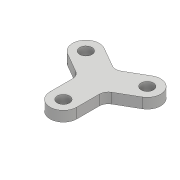
# Autodesk Inventor part: carrier2
Saved by Autodesk Inventor 2018 (Build 220112000, 112)
## iProperties
Created: 2019-12-31
Part Number: carrier2
Material: 一般
Document SubType Name: Modeling
Designer: louis
Density: 1 g/cm^3
Appearance: 預設
Author: louis
Autodesk Inventor part; units mm, degrees
ref_plane "YZ Plane" through (0, 0, 0) normal (1, 0, 0) x (0, 1, 0)
ref_plane "XZ Plane" through (0, 0, 0) normal (0, 1, 0) x (-1, 0, 0)
ref_plane "XY Plane" through (0, 0, 0) normal (0, 0, 1) x (1, 0, 0)
sketch "草圖1" plane through (0, 0, 0) normal (0, 0, 1) x (1, 0, 0)
  line L0 (0, 0) -> (-29.8779, 17.25) construction
  line L1 (0, 0) -> (0, -34.5) construction
  circle A0 centre (29.8779, 17.25) radius 6
  circle A1 centre (0, -34.5) radius 6
  circle A2 centre (-29.8779, 17.25) radius 6
  line L2 (-23.3779, 28.5083) -> (-4.3253, 17.5083)
  arc A3 (-4.3253, 17.5083) -> (4.3253, 17.5083) centre (0, 25) ccw
  line L3 (4.3253, 17.5083) -> (23.3779, 28.5083)
  line L4 (23.3779, 28.5083) -> (23.3779, 28.5083)
  arc A4 (36.3779, 5.9917) -> (23.3779, 28.5083) centre (29.8779, 17.25) ccw
  line L5 (36.3779, 5.9917) -> (17.3253, -5.0083)
  arc A5 (17.3253, -5.0083) -> (13, -12.5) centre (21.6506, -12.5) ccw
  line L6 (13, -12.5) -> (13, -34.5)
  arc A6 (-13, -34.5) -> (13, -34.5) centre (0, -34.5) ccw
  line L7 (-13, -34.5) -> (-13, -12.5)
  arc A7 (-13, -12.5) -> (-17.3253, -5.0083) centre (-21.6506, -12.5) ccw
  line L8 (-17.3253, -5.0083) -> (-36.3779, 5.9917)
  arc A8 (-23.3779, 28.5083) -> (-36.3779, 5.9917) centre (-29.8779, 17.25) ccw
  line L9 (0, 0) -> (29.8779, 17.25) construction
  dimension "d0" = 34.5
  dimension "d4" = 120
  dimension "d5" = 34.5
  dimension "d6" = 12
  dimension "d7" = 12
  dimension "d8" = 12
  dimension "d9" = 7
  dimension "d10" = 7
  dimension "d11" = 7
  dimension "d12" = 34.5
  dimension "d13" = 120
  dimension "d35" = 25
  constraints: 20 end point, 12 point on circle, 12 tangent, 9 centre point, 4 equal length, 4 parallel, 3 concentric, 2 coincident, 1 vertical
  measures "d0" distance of L0.start L0.end
  measures "d5" distance of L0.start L1.end
  measures "d6" diameter of A2
  measures "d7" diameter of A0
  measures "d8" diameter of A1
  measures "d9" radial gap between concentric circles of A8 A2
  measures "d10" radial gap between concentric circles of A4 A0
  measures "d11" radial gap between concentric circles of A6 A1
  measures "d12" distance of L0.start L9.end
  measures "d35" distance of L0.start A3.centre
extrude "擠出1" add sketch "草圖1" along normal blind 10
equation "\"d10\" = d9"
equation "\"d11\" = d9"
